Autodesk Fusion 360 part; units mm, degrees
(part 6 of 7)
sketch "Provisional CO PCB left-face seat sketch" plane through (0, 0, 24.5) normal (0, 0, 1) x (1, 0, 0) in component "Chamber / A3 top manifold with serial return"
  line L0 (4.9, 133) -> (8.95, 133)
  line L1 (8.95, 133) -> (8.95, 135)
  line L2 (8.95, 135) -> (4.9, 135)
  line L3 (4.9, 135) -> (4.9, 133)
  dimension "d2293" = 4.9
  dimension "d2294" = 133
  dimension "d2295" = 4.05
  dimension "d2296" = 2
  constraint horizontal L0
  constraint vertical L1
  constraint horizontal L2
  constraint vertical L3
  measures "d2293" horizontal distance of origin L0.start
  measures "d2294" vertical distance of origin L0.start
  measures "d2295" horizontal distance of L0.start L0.end
  measures "d2296" vertical distance of L0.end L1.end
extrude "Provisional CO PCB left-face seat" add sketch "Provisional CO PCB left-face seat sketch" along normal blind 2 bodies 74 in component "Chamber / A3 top manifold with serial return"
ref_plane "WorkPlane39" through (0, 0, 8) normal (0, 0, 1) x (1, 0, 0) in component "Chamber / A3 top manifold with serial return"
sketch "Provisional CO PCB left-face seat sketch (1)" plane through (0, 0, 8) normal (0, 0, 1) x (1, 0, 0) in component "Chamber / A3 top manifold with serial return"
  line L0 (4.9, 155) -> (8.95, 155)
  line L1 (8.95, 155) -> (8.95, 157)
  line L2 (8.95, 157) -> (4.9, 157)
  line L3 (4.9, 157) -> (4.9, 155)
  dimension "d2301" = 4.9
  dimension "d2302" = 155
  dimension "d2303" = 4.05
  dimension "d2304" = 2
  constraint horizontal L0
  constraint vertical L1
  constraint horizontal L2
  constraint vertical L3
  measures "d2301" horizontal distance of origin L0.start
  measures "d2302" vertical distance of origin L0.start
  measures "d2303" horizontal distance of L0.start L0.end
  measures "d2304" vertical distance of L0.end L1.end
extrude "Provisional CO PCB left-face seat (1)" add sketch "Provisional CO PCB left-face seat sketch (1)" along normal blind 2 bodies 74 in component "Chamber / A3 top manifold with serial return"
ref_plane "WorkPlane40" through (0, 0, 4.9) normal (0, 0, 1) x (1, 0, 0) in component "Chamber / A3 top manifold with serial return"
sketch "Provisional CO front-edge seat sketch" plane through (0, 0, 4.9) normal (0, 0, 1) x (1, 0, 0) in component "Chamber / A3 top manifold with serial return"
  line L0 (8.75, 133) -> (10.75, 133)
  line L1 (10.75, 133) -> (10.75, 135)
  line L2 (10.75, 135) -> (8.75, 135)
  line L3 (8.75, 135) -> (8.75, 133)
  dimension "d2309" = 8.75
  dimension "d2310" = 133
  dimension "d2311" = 2
  dimension "d2312" = 2
  constraint horizontal L0
  constraint vertical L1
  constraint horizontal L2
  constraint vertical L3
  measures "d2309" horizontal distance of origin L0.start
  measures "d2310" vertical distance of origin L0.start
  measures "d2311" horizontal distance of L0.start L0.end
  measures "d2312" vertical distance of L0.end L1.end
extrude "Provisional CO front-edge seat" add sketch "Provisional CO front-edge seat sketch" along normal blind 0.5 bodies 74 in component "Chamber / A3 top manifold with serial return"
ref_plane "WorkPlane41" through (0, 0, 6) normal (0, 0, 1) x (1, 0, 0) in component "Chamber / A3 top manifold with serial return"
sketch "Provisional CO upper corner keeper sketch" plane through (0, 0, 6) normal (0, 0, 1) x (1, 0, 0) in component "Chamber / A3 top manifold with serial return"
  line L0 (10.7, 155.5) -> (12.7, 155.5)
  line L1 (12.7, 155.5) -> (12.7, 159.5)
  line L2 (12.7, 159.5) -> (10.7, 159.5)
  line L3 (10.7, 159.5) -> (10.7, 155.5)
  dimension "d2317" = 10.7
  dimension "d2318" = 155.5
  dimension "d2319" = 2
  dimension "d2320" = 4
  constraint horizontal L0
  constraint vertical L1
  constraint horizontal L2
  constraint vertical L3
  measures "d2317" horizontal distance of origin L0.start
  measures "d2318" vertical distance of origin L0.start
  measures "d2319" horizontal distance of L0.start L0.end
  measures "d2320" vertical distance of L0.end L1.end
extrude "Provisional CO upper corner keeper" add sketch "Provisional CO upper corner keeper sketch" along normal blind 2 bodies 74 in component "Chamber / A3 top manifold with serial return"
ref_plane "WorkPlane42" through (0, 0, 25) normal (0, 0, 1) x (1, 0, 0) in component "Chamber / A3 top manifold with serial return"
sketch "Provisional CO lower corner keeper sketch" plane through (0, 0, 25) normal (0, 0, 1) x (1, 0, 0) in component "Chamber / A3 top manifold with serial return"
  line L0 (10.7, 131.5) -> (12.7, 131.5)
  line L1 (12.7, 131.5) -> (12.7, 134.3)
  line L2 (12.7, 134.3) -> (10.7, 134.3)
  line L3 (10.7, 134.3) -> (10.7, 131.5)
  dimension "d2325" = 10.7
  dimension "d2326" = 131.5
  dimension "d2327" = 2
  dimension "d2328" = 2.8
  constraint horizontal L0
  constraint vertical L1
  constraint horizontal L2
  constraint vertical L3
  measures "d2325" horizontal distance of origin L0.start
  measures "d2326" vertical distance of origin L0.start
  measures "d2327" horizontal distance of L0.start L0.end
  measures "d2328" vertical distance of L0.end L1.end
extrude "Provisional CO lower corner keeper" add sketch "Provisional CO lower corner keeper sketch" along normal blind 2 bodies 74 in component "Chamber / A3 top manifold with serial return"
ref_plane "WorkPlane43" through (0, 0, 4.9) normal (0, 0, 1) x (1, 0, 0) in component "Chamber / A3 top manifold with serial return"
sketch "Provisional MD62 front end-contact sketch" plane through (0, 0, 4.9) normal (0, 0, 1) x (1, 0, 0) in component "Chamber / A3 top manifold with serial return"
  line L0 (21.5, 164) -> (23.5, 164)
  line L1 (23.5, 164) -> (23.5, 166)
  line L2 (23.5, 166) -> (21.5, 166)
  line L3 (21.5, 166) -> (21.5, 164)
  dimension "d2333" = 21.5
  dimension "d2334" = 164
  dimension "d2335" = 2
  dimension "d2336" = 2
  constraint horizontal L0
  constraint vertical L1
  constraint horizontal L2
  constraint vertical L3
  measures "d2333" horizontal distance of origin L0.start
  measures "d2334" vertical distance of origin L0.start
  measures "d2335" horizontal distance of L0.start L0.end
  measures "d2336" vertical distance of L0.end L1.end
extrude "Provisional MD62 front end-contact" add sketch "Provisional MD62 front end-contact sketch" along normal blind 3.1 bodies 74 in component "Chamber / A3 top manifold with serial return"
ref_plane "WorkPlane7" through (0, 0, 27.3) normal (0, 0, 1) x (1, 0, 0) in component "Chamber / A3 four-screw service lid"
sketch "Sketch7" plane through (0, 0, 27.3) normal (0, 0, 1) x (1, 0, 0) in component "Chamber / A3 four-screw service lid"
  line L0 (21.5, 164) -> (23.5, 164)
  line L1 (23.5, 164) -> (23.5, 166)
  line L2 (23.5, 166) -> (21.5, 166)
  line L3 (21.5, 166) -> (21.5, 164)
  dimension "d2341" = 21.5
  dimension "d2342" = 164
  dimension "d2343" = 2
  dimension "d2344" = 2
  constraint horizontal L0
  constraint vertical L1
  constraint horizontal L2
  constraint vertical L3
  measures "d2341" horizontal distance of origin L0.start
  measures "d2342" vertical distance of origin L0.start
  measures "d2343" horizontal distance of L0.start L0.end
  measures "d2344" vertical distance of L0.end L1.end
extrude "Provisional MD62 rear end-stop — 0.3 mm gap" add sketch "Sketch7" along normal blind 8.8 bodies 75 in component "Chamber / A3 four-screw service lid"
ref_plane "WorkPlane44" through (0, 0, 4.9) normal (0, 0, 1) x (1, 0, 0) in component "Chamber / A3 top manifold with serial return"
sketch "Provisional MD62 front end-contact sketch (1)" plane through (0, 0, 4.9) normal (0, 0, 1) x (1, 0, 0) in component "Chamber / A3 top manifold with serial return"
  line L0 (21.5, 169.8) -> (23.5, 169.8)
  line L1 (23.5, 169.8) -> (23.5, 171.8)
  line L2 (23.5, 171.8) -> (21.5, 171.8)
  line L3 (21.5, 171.8) -> (21.5, 169.8)
  dimension "d2349" = 21.5
  dimension "d2350" = 169.8
  dimension "d2351" = 2
  dimension "d2352" = 2
  constraint horizontal L0
  constraint vertical L1
  constraint horizontal L2
  constraint vertical L3
  measures "d2349" horizontal distance of origin L0.start
  measures "d2350" vertical distance of origin L0.start
  measures "d2351" horizontal distance of L0.start L0.end
  measures "d2352" vertical distance of L0.end L1.end
extrude "Provisional MD62 front end-contact (1)" add sketch "Provisional MD62 front end-contact sketch (1)" along normal blind 3.1 bodies 74 in component "Chamber / A3 top manifold with serial return"
ref_plane "WorkPlane8" through (0, 0, 27.3) normal (0, 0, 1) x (1, 0, 0) in component "Chamber / A3 four-screw service lid"
sketch "Sketch8" plane through (0, 0, 27.3) normal (0, 0, 1) x (1, 0, 0) in component "Chamber / A3 four-screw service lid"
  line L0 (21.5, 169.8) -> (23.5, 169.8)
  line L1 (23.5, 169.8) -> (23.5, 171.8)
  line L2 (23.5, 171.8) -> (21.5, 171.8)
  line L3 (21.5, 171.8) -> (21.5, 169.8)
  dimension "d2357" = 21.5
  dimension "d2358" = 169.8
  dimension "d2359" = 2
  dimension "d2360" = 2
  constraint horizontal L0
  constraint vertical L1
  constraint horizontal L2
  constraint vertical L3
  measures "d2357" horizontal distance of origin L0.start
  measures "d2358" vertical distance of origin L0.start
  measures "d2359" horizontal distance of L0.start L0.end
  measures "d2360" vertical distance of L0.end L1.end
extrude "Provisional MD62 rear end-stop — 0.3 mm gap (1)" add sketch "Sketch8" along normal blind 8.8 bodies 75 in component "Chamber / A3 four-screw service lid"
ref_plane "WorkPlane45" through (0, 0, 4.9) normal (0, 0, 1) x (1, 0, 0) in component "Chamber / A3 top manifold with serial return"
sketch "Provisional MD62 lateral guide sketch" plane through (0, 0, 4.9) normal (0, 0, 1) x (1, 0, 0) in component "Chamber / A3 top manifold with serial return"
  line L0 (16.7, 163.5) -> (18.7, 163.5)
  line L1 (18.7, 163.5) -> (18.7, 171.5)
  line L2 (18.7, 171.5) -> (16.7, 171.5)
  line L3 (16.7, 171.5) -> (16.7, 163.5)
  dimension "d2365" = 16.7
  dimension "d2366" = 163.5
  dimension "d2367" = 2
  dimension "d2368" = 8
  constraint horizontal L0
  constraint vertical L1
  constraint horizontal L2
  constraint vertical L3
  measures "d2365" horizontal distance of origin L0.start
  measures "d2366" vertical distance of origin L0.start
  measures "d2367" horizontal distance of L0.start L0.end
  measures "d2368" vertical distance of L0.end L1.end
extrude "Provisional MD62 lateral guide" add sketch "Provisional MD62 lateral guide sketch" along normal blind 5.1 bodies 74 in component "Chamber / A3 top manifold with serial return"
ref_plane "WorkPlane46" through (0, 0, 4.9) normal (0, 0, 1) x (1, 0, 0) in component "Chamber / A3 top manifold with serial return"
sketch "Provisional MD62 lateral guide sketch (1)" plane through (0, 0, 4.9) normal (0, 0, 1) x (1, 0, 0) in component "Chamber / A3 top manifold with serial return"
  line L0 (33.3, 163.5) -> (35.3, 163.5)
  line L1 (35.3, 163.5) -> (35.3, 171.5)
  line L2 (35.3, 171.5) -> (33.3, 171.5)
  line L3 (33.3, 171.5) -> (33.3, 163.5)
  dimension "d2373" = 33.3
  dimension "d2374" = 163.5
  dimension "d2375" = 2
  dimension "d2376" = 8
  constraint horizontal L0
  constraint vertical L1
  constraint horizontal L2
  constraint vertical L3
  measures "d2373" horizontal distance of origin L0.start
  measures "d2374" vertical distance of origin L0.start
  measures "d2375" horizontal distance of L0.start L0.end
  measures "d2376" vertical distance of L0.end L1.end
extrude "Provisional MD62 lateral guide (1)" add sketch "Provisional MD62 lateral guide sketch (1)" along normal blind 5.1 bodies 74 in component "Chamber / A3 top manifold with serial return"
ref_plane "WorkPlane47" through (0, 0, 4.9) normal (0, 0, 1) x (1, 0, 0) in component "Chamber / A3 top manifold with serial return"
sketch "Provisional humidity PCB foot sketch" plane through (0, 0, 4.9) normal (0, 0, 1) x (1, 0, 0) in component "Chamber / A3 top manifold with serial return"
  line L0 (54, 164) -> (56, 164)
  line L1 (56, 164) -> (56, 166)
  line L2 (56, 166) -> (54, 166)
  line L3 (54, 166) -> (54, 164)
  dimension "d2381" = 54
  dimension "d2382" = 164
  dimension "d2383" = 2
  dimension "d2384" = 2
  constraint horizontal L0
  constraint vertical L1
  constraint horizontal L2
  constraint vertical L3
  measures "d2381" horizontal distance of origin L0.start
  measures "d2382" vertical distance of origin L0.start
  measures "d2383" horizontal distance of L0.start L0.end
  measures "d2384" vertical distance of L0.end L1.end
extrude "Provisional humidity PCB foot" add sketch "Provisional humidity PCB foot sketch" along normal blind 1.1 bodies 74 in component "Chamber / A3 top manifold with serial return"
ref_plane "WorkPlane48" through (0, 0, 4.9) normal (0, 0, 1) x (1, 0, 0) in component "Chamber / A3 top manifold with serial return"
sketch "Provisional humidity PCB foot sketch (1)" plane through (0, 0, 4.9) normal (0, 0, 1) x (1, 0, 0) in component "Chamber / A3 top manifold with serial return"
  line L0 (67, 172) -> (69, 172)
  line L1 (69, 172) -> (69, 174)
  line L2 (69, 174) -> (67, 174)
  line L3 (67, 174) -> (67, 172)
  dimension "d2389" = 67
  dimension "d2390" = 172
  dimension "d2391" = 2
  dimension "d2392" = 2
  constraint horizontal L0
  constraint vertical L1
  constraint horizontal L2
  constraint vertical L3
  measures "d2389" horizontal distance of origin L0.start
  measures "d2390" vertical distance of origin L0.start
  measures "d2391" horizontal distance of L0.start L0.end
  measures "d2392" vertical distance of L0.end L1.end
extrude "Provisional humidity PCB foot (1)" add sketch "Provisional humidity PCB foot sketch (1)" along normal blind 1.1 bodies 74 in component "Chamber / A3 top manifold with serial return"
ref_plane "WorkPlane49" through (0, 0, 7.9) normal (0, 0, 1) x (1, 0, 0) in component "Chamber / A3 top manifold with serial return"
sketch "Provisional humidity corner keeper sketch" plane through (0, 0, 7.9) normal (0, 0, 1) x (1, 0, 0) in component "Chamber / A3 top manifold with serial return"
  line L0 (68, 164) -> (70.6, 164)
  line L1 (70.6, 164) -> (70.6, 166)
  line L2 (70.6, 166) -> (68, 166)
  line L3 (68, 166) -> (68, 164)
  dimension "d2397" = 68
  dimension "d2398" = 164
  dimension "d2399" = 2.6
  dimension "d2400" = 2
  constraint horizontal L0
  constraint vertical L1
  constraint horizontal L2
  constraint vertical L3
  measures "d2397" horizontal distance of origin L0.start
  measures "d2398" vertical distance of origin L0.start
  measures "d2399" horizontal distance of L0.start L0.end
  measures "d2400" vertical distance of L0.end L1.end
extrude "Provisional humidity corner keeper" add sketch "Provisional humidity corner keeper sketch" along normal blind 2 bodies 74 in component "Chamber / A3 top manifold with serial return"
component "01 Shape A housing" placed x (1, 0, 0) y (0, 1, 0) z (0, 0, 1) at (0, 0, 0)
component "02 Single rear cover" placed x (1, 0, 0) y (0, 1, 0) z (0, 0, 1) at (0, 0, 0)
component "03 Guition factory casing — measured envelope" placed x (1, 0, 0) y (0, 1, 0) z (0, 0, 1) at (0, 0, 0)
component "04 Guition front glass — drawing reference" placed x (1, 0, 0) y (0, 1, 0) z (0, 0, 1) at (0, 0, 0)
component "05 Active 4.3 inch screen" placed x (1, 0, 0) y (0, 1, 0) z (0, 0, 1) at (0, 0, 0)
component "06 Guition PCB and connectors — illustrative detail" placed x (1, 0, 0) y (0, 1, 0) z (0, 0, 1) at (0, 0, 0)
component "M3 x 8 button screw — GEN-M3-BHCS-L8-AF2" placed x (1, 0, 0) y (0, 1, 0) z (0, 0, 1) at (8, 8, 41.35)
component "M3 insert OD4.2 x5 — GEN-M3-HEATSET-OD4.2-L5" placed x (1, 0, 0) y (0, 1, 0) z (0, 0, 1) at (8, 8, 39)
component "Carrier / removable electronics tray" placed x (1, 0, 0) y (0, 1, 0) z (0, 0, 1) at (0, 0, 0)
component "Carrier / future PCB allocation — layout pending" placed x (1, 0, 0) y (0, 1, 0) z (0, 0, 1) at (0, 0, 0)
component "M2 x 7 socket_cap screw — GEN-M2-SHCS-L7-AF1.5" placed x (1, 0, 0) y (0, 1, 0) z (0, 0, 1) at (76, 28, 22.1)
component "M2 insert OD3.2 x4 — GEN-M2-HEATSET-OD3.2-L4" placed x (1, 0, 0) y (0, 1, 0) z (0, 0, 1) at (76, 28, 18.5)
component "Display / lower rear-release retainer" placed x (1, 0, 0) y (0, 1, 0) z (0, 0, 1) at (0, 0, 0)
component "Display / upper rear-release retainer" placed x (1, 0, 0) y (0, 1, 0) z (0, 0, 1) at (0, 0, 0)
component "M2 x 5 socket_cap screw — GEN-M2-SHCS-L5-AF1.5" placed x (1, 0, 0) y (0, 1, 0) z (0, 0, 1) at (69, 12.3, 20.5)
component "Battery / FMA protected holder - owner-measured envelope" placed x (1, 0, 0) y (0, 1, 0) z (0, 0, 1) at (0, 0, 0)
component "Battery / 18650 cell A - owner-rated 3400 mAh" placed x (1, 0, 0) y (0, 1, 0) z (0, 0, 1) at (0, 0, 0)
component "Battery / 18650 cell B - owner-rated 3400 mAh" placed x (1, 0, 0) y (0, 1, 0) z (0, 0, 1) at (0, 0, 0)
component "Battery / red RCY disconnect body - provisional reference" placed x (1, 0, 0) y (0, 1, 0) z (0, 0, 1) at (0, 0, 0)
component "Battery / red RCY disconnect mate - provisional reference" placed x (1, 0, 0) y (0, 1, 0) z (0, 0, 1) at (0, 0, 0)
component "Controls / left 1NO button body" placed x (1, 0, 0) y (0, 1, 0) z (0, 0, 1) at (0, 0, 0)
component "Controls / left momentary power cap" placed x (1, 0, 0) y (0, 1, 0) z (0, 0, 1) at (0, 0, 0)
component "Controls / button retaining nut reference" placed x (1, 0, 0) y (0, 1, 0) z (0, 0, 1) at (0, 0, 0)
component "USB A3 — tiny flush metal bezel and hidden flange" placed x (1, 0, 0) y (0, 1, 0) z (0, 0, 1) at (0, 0, 0)
component "USB A3 — removable printed support frame" placed x (1, 0, 0) y (0, 1, 0) z (0, 0, 1) at (0, 0, 0)
component "USB A3 — hidden metal retaining bridge" placed x (1, 0, 0) y (0, 1, 0) z (0, 0, 1) at (0, 0, 0)
component "USB A3 — supported 0.60 mm daughterboard provisional" placed x (1, 0, 0) y (0, 1, 0) z (0, 0, 1) at (0, 0, 0)
component "USB A3 — GCT USB4720 shell drawing reconstruction" placed x (1, 0, 0) y (0, 1, 0) z (0, 0, 1) at (0, 0, 0)
component "USB A3 — tongue and rear insulator reference" placed x (1, 0, 0) y (0, 1, 0) z (0, 0, 1) at (0, 0, 0)
component "USB A3 — GCT LIM gasket nominal reference" placed x (1, 0, 0) y (0, 1, 0) z (0, 0, 1) at (0, 0, 0)
component "USB A3 — illustrative contact stripes" placed x (1, 0, 0) y (0, 1, 0) z (0, 0, 1) at (0, 0, 0)
component "Chamber / A3 top manifold with serial return" placed x (1, 0, 0) y (0, 1, 0) z (0, 0, 1) at (0, 0, 0)
component "Chamber / A3 four-screw service lid" placed x (1, 0, 0) y (0, 1, 0) z (0, 0, 1) at (0, 0, 0)
component "Chamber / AO2 hand-tight adapter reference" placed x (1, 0, 0) y (0, 1, 0) z (0, 0, 1) at (0, 0, 0)
component "Sensor / AO2 dry body with wetted threaded nose" placed x (1, 0, 0) y (0, 1, 0) z (0, 0, 1) at (0, 0, 0)
component "Sensor / AO2 cable connector allowance" placed x (1, 0, 0) y (0, 1, 0) z (0, 0, 1) at (0, 0, 0)
component "Sensor / ZE07-CO drawing-derived assembly" placed x (1, 0, 0) y (0, 1, 0) z (0, 0, 1) at (0, 0, 0)
component "Sensor / MD62 body and full-length lead references" placed x (1, 0, 0) y (0, 1, 0) z (0, 0, 1) at (0, 0, 0)
component "Sensor / GYBMEP humidity breakout reference" placed x (1, 0, 0) y (0, 1, 0) z (0, 0, 1) at (0, 0, 0)
component "Gas / Viewer-left inlet fitting reference" placed x (1, 0, 0) y (0, 1, 0) z (0, 0, 1) at (0, 0, 0)
component "Gas / Viewer-right exhaust fitting reference" placed x (1, 0, 0) y (0, 1, 0) z (0, 0, 1) at (0, 0, 0)
component "Chamber / AO2 face-seal allowance" placed x (1, 0, 0) y (0, 1, 0) z (0, 0, 1) at (0, 0, 0)
component "Chamber / sealed harness feedthrough allowance" placed x (1, 0, 0) y (0, 1, 0) z (0, 0, 1) at (0, 0, 0)
component "M3 x 8 button screw — GEN-M3-BHCS-L8-AF2" placed x (1, 0, 0) y (0, 1, 0) z (0, 0, 1) at (77, 8, 41.35)
component "M3 x 8 button screw — GEN-M3-BHCS-L8-AF2" placed x (1, 0, 0) y (0, 1, 0) z (0, 0, 1) at (8, 172, 41.35)
component "M3 x 8 button screw — GEN-M3-BHCS-L8-AF2" placed x (1, 0, 0) y (0, 1, 0) z (0, 0, 1) at (77, 172, 41.35)
component "M3 insert OD4.2 x5 — GEN-M3-HEATSET-OD4.2-L5" placed x (1, 0, 0) y (0, 1, 0) z (0, 0, 1) at (77, 8, 39)
component "M3 insert OD4.2 x5 — GEN-M3-HEATSET-OD4.2-L5" placed x (1, 0, 0) y (0, 1, 0) z (0, 0, 1) at (8, 172, 39)
component "M3 insert OD4.2 x5 — GEN-M3-HEATSET-OD4.2-L5" placed x (1, 0, 0) y (0, 1, 0) z (0, 0, 1) at (77, 172, 39)
component "M2 x 7 socket_cap screw — GEN-M2-SHCS-L7-AF1.5" placed x (1, 0, 0) y (0, 1, 0) z (0, 0, 1) at (54.8, 114, 22.1)
component "M2 insert OD3.2 x4 — GEN-M2-HEATSET-OD3.2-L4" placed x (1, 0, 0) y (0, 1, 0) z (0, 0, 1) at (54.8, 114, 18.5)
component "M2 x 5 socket_cap screw — GEN-M2-SHCS-L5-AF1.5" placed x (1, 0, 0) y (0, 1, 0) z (0, 0, 1) at (10.5, 126, 20.5)
component "M2 insert OD3.2 x4 — GEN-M2-HEATSET-OD3.2-L4" placed x (1, 0, 0) y (0, 1, 0) z (0, 0, 1) at (69, 12.3, 18.5)
component "M2 insert OD3.2 x4 — GEN-M2-HEATSET-OD3.2-L4" placed x (1, 0, 0) y (0, 1, 0) z (0, 0, 1) at (10.5, 126, 18.5)
component "M2 x 5 socket_cap screw — GEN-M2-SHCS-L5-AF1.5" placed x (1, 0, 0) y (0, 1, 0) z (0, 0, 1) at (33.25, 18.25, 33.2)
component "M2 x 5 socket_cap screw — GEN-M2-SHCS-L5-AF1.5" placed x (1, 0, 0) y (0, 1, 0) z (0, 0, 1) at (51.75, 18.25, 33.2)
component "M2 insert OD3.2 x4 — GEN-M2-HEATSET-OD3.2-L4" placed x (1, 0, 0) y (0, 1, 0) z (0, 0, 1) at (33.25, 18.25, 31.2)
component "M2 insert OD3.2 x4 — GEN-M2-HEATSET-OD3.2-L4" placed x (1, 0, 0) y (0, 1, 0) z (0, 0, 1) at (51.75, 18.25, 31.2)
component "M2 x 5 socket_cap screw — GEN-M2-SHCS-L5-AF1.5" placed x (1, 0, 0) y (0, 1, 0) z (0, 0, 1) at (18, 159, 38)
component "M2 x 5 socket_cap screw — GEN-M2-SHCS-L5-AF1.5" placed x (1, 0, 0) y (0, 1, 0) z (0, 0, 1) at (30.5, 135, 38)
component "M2 x 5 socket_cap screw — GEN-M2-SHCS-L5-AF1.5" placed x (1, 0, 0) y (0, 1, 0) z (0, 0, 1) at (17, 172.2, 38)
component "M2 x 5 socket_cap screw — GEN-M2-SHCS-L5-AF1.5" placed x (1, 0, 0) y (0, 1, 0) z (0, 0, 1) at (68, 172.2, 38)
component "M2 insert OD3.2 x4 — GEN-M2-HEATSET-OD3.2-L4" placed x (1, 0, 0) y (0, 1, 0) z (0, 0, 1) at (18, 159, 36)
component "M2 insert OD3.2 x4 — GEN-M2-HEATSET-OD3.2-L4" placed x (1, 0, 0) y (0, 1, 0) z (0, 0, 1) at (30.5, 135, 36)
component "M2 insert OD3.2 x4 — GEN-M2-HEATSET-OD3.2-L4" placed x (1, 0, 0) y (0, 1, 0) z (0, 0, 1) at (17, 172.2, 36)
component "M2 insert OD3.2 x4 — GEN-M2-HEATSET-OD3.2-L4" placed x (1, 0, 0) y (0, 1, 0) z (0, 0, 1) at (68, 172.2, 36)
component "Trimix_Enclosure_A3 v2" placed x (1, 0, 0) y (0, 1, 0) z (0, 0, 1) at (0, 0, 0) in component "03 Guition factory casing — measured envelope"
component "01 Shape A housing" placed x (1, 0, 0) y (0, 1, 0) z (0, 0, 1) at (0, 0, 0) in component "Chamber / A3 four-screw service lid"
equation "CaseWidth = 85 mm" comment "Accepted maximum starting width; test narrower packaging"
equation "CaseHeight = 180 mm" comment "Taller top sampling pod accepted for a slimmer grip"
equation "CaseDepth = 43 mm" comment "Body including flush rear screw heads"
equation "Wall = 2.4 mm" comment "Nominal printed structural wall, selected sections minimum2mm"
equation "RearInset = 0.25 mm" comment "Small rearward taper per side; Shape A straight-sided intent"
equation "CornerRadius = 8 mm" comment "Restrained Shape A outline rounds"
equation "Cover = 2.4 mm" comment "Single rear cover nominal thickness"
equation "CoverGap = 0.2 mm" comment "Assembly gap, not a qualified weather seal"
equation "DisplayWidth = 69.3 mm" comment "Owner measured retained factory casing"
equation "DisplayHeight = 116.8 mm" comment "Owner measured retained factory casing"
equation "DisplayDepth = 13.7 mm" comment "Owner measured with factory back removed"
equation "DisplayX = ( CaseWidth - DisplayWidth ) / 2" comment "Purchased assembly remains centred"
equation "DisplayY = 5.2 mm" comment "Fixed lower front border"
equation "DisplayFront = 0.4 mm" comment "Front recess"
equation "DisplayFit = 0.4 mm" comment "Provisional fit clearance per side"
equation "GlassWidth = 66.8 mm" comment "Manufacturer drawing reference"
equation "GlassHeight = 114.4 mm" comment "Manufacturer drawing reference"
equation "ActiveWidth = 56.16 mm" comment "Manufacturer active-area reference"
equation "ActiveHeight = 93.60 mm" comment "Manufacturer active-area reference"
equation "HolderWidth = 42 mm" comment "Owner measured occupied protected FMA holder"
equation "HolderHeight = 80.4 mm" comment "Owner measured occupied protected FMA holder"
equation "HolderDepth = 20.35 mm" comment "Owner measured occupied protected FMA holder"
equation "HolderX = 5.4 mm" comment "Right-hand rear battery bay"
equation "HolderY = 27 mm" comment "Clear bottom USB cartridge and cable region"
equation "HolderZ = 16.5 mm" comment "2.4mm beyond maximum purchased display depth"
equation "PcbX = 50.4 mm" comment "PCB strip beside holder; no stack behind battery"
equation "PcbY = 21 mm" comment "Low end of PCB strip"
equation "PcbWidth = CaseWidth - PcbX - 4.6 mm" comment "Future PCB allocation; routed fit pending"
equation "PcbHeight = 99 mm" comment "Future PCB strip height before button notch"
equation "PcbZ = 20.5 mm" comment "PCB front plane; carrier and support below"
equation "ButtonY = 113 mm" comment "Viewer-left button above pack; PCB notch"
equation "ButtonZ = 31 mm" comment "Unmeasured button assembly depth centre"
equation "UsbX = CaseWidth / 2" comment "Centred bottom USB socket"
equation "UsbZ = 26 mm" comment "Bottom USB socket depth centre"
equation "GasY = CaseHeight - 17.5 mm" comment "Upper opposed sample ports"
equation "GasZ = 22 mm" comment "Sample port depth centre"
equation "d39 = CaseWidth"
equation "d40 = CaseHeight"
equation "d41 = CaseDepth - Cover"
equation "d43 = RearInset"
equation "d44 = RearInset"
equation "d45 = CaseWidth - 2 * RearInset"
equation "d46 = CaseHeight - 2 * RearInset"
equation "d48 = CornerRadius"
equation "d51 = Wall"
equation "d52 = Wall"
equation "d53 = CaseWidth - 2 * Wall"
equation "d54 = CaseHeight - 2 * Wall"
equation "d55 = CaseDepth"
equation "d58 = CornerRadius - Wall"
equation "d59 = Wall"
equation "d61 = Wall"
equation "d63 = CaseWidth - 2 * Wall"
equation "d64 = CaseHeight - Wall - 128 mm"
equation "d65 = CaseDepth"
equation "d68 = CornerRadius - Wall"
equation "d71 = DisplayX - DisplayFit"
equation "d72 = DisplayY - DisplayFit"
equation "d73 = DisplayWidth + 2 * DisplayFit"
equation "d74 = DisplayHeight + 2 * DisplayFit"
equation "d81 = -( -( GasZ ) )"
equation "d82 = GasY"
equation "d84 = CaseWidth + 2 mm"
equation "d86 = CaseWidth - Wall - 1 mm"
equation "d88 = -( -( ButtonZ ) )"
equation "d89 = ButtonY"
equation "d91 = Wall + 2 mm"
equation "d93 = CaseDepth - Cover + CoverGap"
equation "d95 = RearInset"
equation "d96 = RearInset"
equation "d97 = CaseWidth - 2 * RearInset"
equation "d98 = CaseHeight - 2 * RearInset"
equation "d99 = Cover - CoverGap"
equation "d102 = CornerRadius"
equation "d105 = DisplayFront"
equation "d107 = DisplayX"
equation "d108 = DisplayY"
equation "d109 = DisplayWidth"
equation "d110 = DisplayHeight"
equation "d111 = DisplayDepth"
equation "d115 = DisplayFront + 3 mm"
equation "d117 = DisplayX + ( DisplayWidth - 65.4 mm ) / 2"
equation "d118 = DisplayY + ( DisplayHeight - 108 mm ) / 2"
equation "d123 = DisplayFront - 0.1 mm"
equation "d125 = DisplayX + ( DisplayWidth - GlassWidth ) / 2"
equation "d126 = DisplayY + ( DisplayHeight - GlassHeight ) / 2"
equation "d127 = GlassWidth"
equation "d128 = GlassHeight"
equation "d131 = DisplayFront"
equation "d133 = DisplayX + ( DisplayWidth - GlassWidth ) / 2"
equation "d134 = DisplayY + ( DisplayHeight - GlassHeight ) / 2"
equation "d135 = GlassWidth"
equation "d136 = GlassHeight"
equation "d139 = DisplayFront - 0.1 mm"
equation "d141 = DisplayX + ( DisplayWidth - ActiveWidth ) / 2"
equation "d142 = DisplayY + ( DisplayHeight - ActiveHeight ) / 2"
equation "d143 = ActiveWidth"
equation "d144 = ActiveHeight"
equation "d147 = DisplayFront"
equation "d149 = DisplayX + ( DisplayWidth - ActiveWidth ) / 2"
equation "d150 = DisplayY + ( DisplayHeight - ActiveHeight ) / 2"
equation "d151 = ActiveWidth"
equation "d152 = ActiveHeight"
equation "d157 = DisplayX + ( DisplayWidth - 65.06 mm ) / 2"
equation "d158 = DisplayY + ( DisplayHeight - 108 mm ) / 2"
equation "d165 = DisplayX + 4.65 mm"
equation "d166 = DisplayY + 7.1 mm"
equation "d172 = DisplayX + 4.65 mm"
equation "d173 = DisplayY + 109.7 mm"
equation "d179 = DisplayX + 64.65 mm"
equation "d180 = DisplayY + 7.1 mm"
equation "d186 = DisplayX + 64.65 mm"
equation "d187 = DisplayY + 109.7 mm"
equation "d193 = DisplayX + 12.15 mm"
equation "d194 = DisplayY + 70.9 mm"
equation "d201 = DisplayX + 44.15 mm"
equation "d202 = DisplayY + 85.9 mm"
equation "d209 = DisplayX + 31.15 mm"
equation "d210 = DisplayY + 74.9 mm"
equation "d217 = DisplayX + 11.15 mm"
equation "d218 = DisplayY + 13.9 mm"
equation "d225 = DisplayX + 21.15 mm"
equation "d226 = DisplayY + 18.9 mm"
equation "d233 = DisplayX + 27.15 mm"
equation "d234 = DisplayY + 4.9 mm"
equation "d241 = DisplayX + 20.15 mm"
equation "d242 = DisplayY + 57.9 mm"
equation "d249 = DisplayX + 49.15 mm"
equation "d250 = DisplayY + 29.9 mm"
equation "d255 = CaseDepth - 13 mm"
equation "d257 = ( 8 mm ) - 3.7 mm"
equation "d258 = Wall - 0.1 mm"
equation "d263 = CaseDepth - 13 mm"
equation "d270 = CaseDepth - 9 mm"
equation "d277 = CaseDepth - 3.8 mm"
equation "d284 = CaseDepth - 3.9 mm"
equation "d291 = CaseDepth - 1.65 mm"
equation "d298 = CaseDepth - 3.9 mm"
equation "d305 = CaseDepth - 13 mm"
equation "d307 = ( CaseWidth - 8 mm ) - 3.7 mm"
equation "d308 = Wall - 0.1 mm"
equation "d313 = CaseDepth - 13 mm"
equation "d315 = CaseWidth - 8 mm"
equation "d320 = CaseDepth - 9 mm"
equation "d322 = CaseWidth - 8 mm"
equation "d327 = CaseDepth - 3.8 mm"
equation "d329 = CaseWidth - 8 mm"
equation "d334 = CaseDepth - 3.9 mm"
equation "d336 = CaseWidth - 8 mm"
equation "d341 = CaseDepth - 1.65 mm"
equation "d343 = CaseWidth - 8 mm"
equation "d348 = CaseDepth - 3.9 mm"
equation "d350 = CaseWidth - 8 mm"
equation "d355 = CaseDepth - 13 mm"
equation "d357 = ( 8 mm ) - 3.7 mm"
equation "d358 = CaseHeight - 11.5 mm"
equation "d363 = CaseDepth - 13 mm"
equation "d366 = CaseHeight - 8 mm"
equation "d370 = CaseDepth - 9 mm"
equation "d373 = CaseHeight - 8 mm"
equation "d377 = CaseDepth - 3.8 mm"
equation "d380 = CaseHeight - 8 mm"
equation "d384 = CaseDepth - 3.9 mm"
equation "d387 = CaseHeight - 8 mm"
equation "d391 = CaseDepth - 1.65 mm"
equation "d394 = CaseHeight - 8 mm"
equation "d398 = CaseDepth - 3.9 mm"
equation "d401 = CaseHeight - 8 mm"
equation "d405 = CaseDepth - 13 mm"
equation "d407 = ( CaseWidth - 8 mm ) - 3.7 mm"
equation "d408 = CaseHeight - 10.5 mm"
equation "d413 = CaseDepth - 13 mm"
equation "d415 = CaseWidth - 8 mm"
equation "d416 = CaseHeight - 8 mm"
equation "d420 = CaseDepth - 9 mm"
equation "d422 = CaseWidth - 8 mm"
equation "d423 = CaseHeight - 8 mm"
equation "d427 = CaseDepth - 3.8 mm"
equation "d429 = CaseWidth - 8 mm"
equation "d430 = CaseHeight - 8 mm"
equation "d434 = CaseDepth - 3.9 mm"
equation "d436 = CaseWidth - 8 mm"
equation "d437 = CaseHeight - 8 mm"
equation "d441 = CaseDepth - 1.65 mm"
equation "d443 = CaseWidth - 8 mm"
equation "d444 = CaseHeight - 8 mm"
equation "d448 = CaseDepth - 3.9 mm"
equation "d450 = CaseWidth - 8 mm"
equation "d451 = CaseHeight - 8 mm"
equation "d493 = CaseDepth - Cover - 2 mm"
equation "d495 = Wall + 0.25 mm"
equation "d501 = CaseDepth - Cover - 2 mm"
equation "d503 = Wall + 0.25 mm"
equation "d509 = CaseDepth - Cover - 2 mm"
equation "d511 = CaseWidth - Wall - 2.25 mm"
equation "d517 = CaseDepth - Cover - 2 mm"
equation "d519 = CaseWidth - Wall - 2.25 mm"
equation "d527 = Wall - 0.1 mm"
equation "d529 = 50.2 mm - Wall + 0.1 mm"
equation "d543 = ( CaseWidth - 9 mm ) - 3.6 mm"
equation "d544 = ( 28 mm ) - 3.6 mm"
equation "d545 = CaseWidth - Wall + 0.1 mm - ( ( CaseWidth - 9 mm ) - 3.6 mm )"
equation "d551 = CaseWidth - 9 mm"
equation "d559 = ( 114 mm ) - 3.6 mm"
equation "d573 = PcbX - 0.2 mm"
equation "d574 = PcbY - 0.5 mm"
equation "d575 = PcbWidth + 0.4 mm"
equation "d576 = PcbHeight + 1 mm"
equation "d579 = PcbZ"
equation "d581 = PcbX"
equation "d582 = PcbY"
equation "d583 = PcbWidth"
equation "d584 = PcbHeight"
equation "d589 = CaseWidth - 26 mm"
equation "d597 = CaseWidth - 9 mm"
equation "d611 = CaseWidth - 26 mm"
equation "d619 = CaseWidth - 9 mm"
equation "d631 = PcbZ + 1.6 mm"
equation "d639 = PcbZ + 1.6 mm"
equation "d647 = PcbZ + 1.6 mm"
equation "d695 = CaseWidth - 17.7 mm"
equation "d703 = CaseWidth - 16 mm"
equation "d710 = CaseWidth - 16 mm"
equation "d717 = DisplayX + 2.65 mm"
equation "d724 = DisplayX + 2.65 mm"
equation "d731 = ( CaseWidth - 16 mm ) - 3.5 mm"
equation "d739 = ( CaseWidth - 16 mm ) - 3 mm"
equation "d740 = DisplayY + 0.5 mm"
equation "d747 = CaseWidth - 16 mm"
equation "d754 = DisplayX - 0.85 mm"
equation "d762 = DisplayX + 0.65 mm"
equation "d763 = DisplayY + DisplayHeight - 2.2 mm"
equation "d770 = DisplayX + 2.65 mm"
equation "d791 = HolderZ"
equation "d793 = HolderX"
equation "d794 = HolderY"
equation "d795 = HolderWidth"
equation "d796 = HolderHeight"
equation "d797 = HolderDepth"
equation "d801 = HolderZ + 1.1 mm"
equation "d803 = HolderX + 1 mm"
equation "d804 = HolderY + 2 mm"
equation "d805 = HolderWidth - 2 mm"
equation "d806 = HolderHeight - 4 mm"
equation "d807 = HolderDepth"
equation "d809 = HolderY + 5 mm"
equation "d811 = HolderX + 10.8 mm"
equation "d812 = -( -( HolderZ + 10.25 mm ) )"
equation "d816 = HolderY + 5 mm"
equation "d818 = HolderX + 31.2 mm"
equation "d819 = -( -( HolderZ + 10.25 mm ) )"
equation "d849 = Wall - 0.1 mm"
equation "d850 = HolderY"
equation "d851 = HolderX - Wall - 0.4 mm"
equation "d852 = HolderHeight"
equation "d857 = Wall - 0.1 mm"
equation "d858 = HolderY - 2.5 mm"
equation "d859 = 50.2 mm - Wall + 0.1 mm"
equation "d865 = Wall - 0.1 mm"
equation "d866 = HolderY + HolderHeight + 0.5 mm"
equation "d867 = 50.2 mm - Wall + 0.1 mm"
equation "d873 = HolderX"
equation "d874 = HolderY"
equation "d876 = HolderHeight"
equation "d879 = HolderZ + HolderDepth + 0.5 mm"
equation "d881 = HolderX"
equation "d882 = HolderY + 12 mm"
equation "d885 = CaseDepth - Cover + CoverGap - HolderZ - HolderDepth - 0.5 mm + 0.2 mm"
equation "d889 = HolderX + HolderWidth - 2 mm"
equation "d890 = HolderY"
equation "d892 = HolderHeight"
equation "d895 = HolderZ + HolderDepth + 0.5 mm"
equation "d897 = HolderX + HolderWidth - 2 mm"
equation "d898 = HolderY + 12 mm"
equation "d901 = CaseDepth - Cover + CoverGap - HolderZ - HolderDepth - 0.5 mm + 0.2 mm"
equation "d903 = CaseWidth - 18 mm"
equation "d905 = -( -( ButtonZ ) )"
equation "d906 = ButtonY"
equation "d910 = CaseWidth"
equation "d912 = -( -( ButtonZ ) )"
equation "d913 = ButtonY"
equation "d917 = CaseWidth - 25 mm"
equation "d919 = -( -( ( ButtonZ - 4 mm ) + ( 8 mm ) ) )"
equation "d920 = ButtonY - 4 mm"
equation "d925 = CaseWidth + 1.3 mm"
equation "d927 = -( -( ButtonZ ) )"
equation "d928 = ButtonY"
equation "d932 = CaseWidth - 4.5 mm"
equation "d934 = -( -( ButtonZ ) )"
equation "d935 = ButtonY"
equation "d939 = CaseWidth - 4.6 mm"
equation "d941 = -( -( ButtonZ ) )"
equation "d942 = ButtonY"
equation "d948 = PcbX - 0.2 mm"
equation "d950 = UsbX + 13.9 mm - PcbX"
equation "d956 = PcbX - 0.2 mm"
equation "d958 = UsbX + 13.9 mm - PcbX"
equation "d962 = CaseDepth - 10 mm"
equation "d969 = CaseDepth - 10 mm"
equation "d972 = CaseHeight - 8 mm"
equation "d976 = CaseDepth - 10 mm"
equation "d978 = CaseWidth - 8 mm"
equation "d983 = CaseDepth - 10 mm"
equation "d985 = CaseWidth - 8 mm"
equation "d986 = CaseHeight - 8 mm"
equation "d992 = UsbX - ( 7 mm )"
equation "d993 = -( -( ( UsbZ - ( 4 mm ) ) + ( 8 mm ) ) )"
equation "d1002 = UsbX - 10 mm"
equation "d1003 = -( -( ( UsbZ - 5 mm ) + ( 11 mm ) ) )"
equation "d1010 = UsbX - 6.5 mm"
equation "d1011 = -( -( ( UsbZ - 3.5 mm ) + ( 7 mm ) ) )"
equation "d1018 = UsbX - ( 4.22 mm )"
equation "d1019 = -( -( ( UsbZ - ( 1.33 mm ) ) + ( 2.66 mm ) ) )"
equation "d1028 = UsbX - ( 4.57 mm )"
equation "d1029 = -( -( ( UsbZ - ( 1.675 mm ) ) + ( 3.35 mm ) ) )"
equation "d1038 = UsbX - ( 4.82 mm )"
equation "d1039 = -( -( ( UsbZ - ( 1.93 mm ) ) + ( 3.86 mm ) ) )"
equation "d1048 = UsbX - ( 4.419249488 mm )"
equation "d1049 = -( -( ( UsbZ - ( 1.529249488 mm ) ) + ( 3.058498976 mm ) ) )"
equation "d1058 = UsbX - ( 4.22 mm )"
equation "d1059 = -( -( ( UsbZ - ( 1.33 mm ) ) + ( 2.66 mm ) ) )"
equation "d1066 = UsbZ - 7 mm"
equation "d1068 = UsbX - 12.9 mm"
equation "d1074 = UsbZ - 5 mm"
equation "d1076 = UsbX - 12.9 mm"
equation "d1082 = UsbZ - 3.2 mm"
equation "d1084 = UsbX - 6.5 mm"
equation "d1090 = UsbZ - 7 mm"
equation "d1092 = UsbX - 9.25 mm"
equation "d1097 = UsbZ + 0.95 mm"
equation "d1099 = UsbX - 9.25 mm"
equation "d1104 = UsbZ - 7 mm"
equation "d1106 = UsbX + 9.25 mm"
equation "d1111 = UsbZ + 0.95 mm"
equation "d1113 = UsbX + 9.25 mm"
equation "d1118 = UsbZ - 5 mm"
equation "d1120 = UsbX - 5.1 mm"
equation "d1126 = UsbZ - 5 mm"
equation "d1128 = UsbX + 3.1 mm"
equation "d1134 = UsbZ - 2.3 mm"
equation "d1136 = UsbX - 5.1 mm"
equation "d1142 = UsbZ + 5.2 mm"
equation "d1144 = UsbX - 12.9 mm"
equation "d1150 = UsbZ + 6 mm"
equation "d1152 = UsbX - 10 mm"
equation "d1158 = UsbZ - 0.3 mm"
equation "d1160 = UsbX - 5.1 mm"
equation "d1166 = UsbZ + 2.3 mm"
equation "d1168 = UsbX - 5.1 mm"
equation "d1174 = UsbZ + 2.3 mm"
equation "d1176 = UsbX + 3.1 mm"
equation "d1182 = UsbZ + 0.3 mm"
equation "d1184 = UsbX - 5.1 mm"
equation "d1190 = UsbZ + 5.1 mm"
equation "d1192 = UsbX - 9.25 mm"
equation "d1197 = UsbZ + 5.1 mm"
equation "d1199 = UsbX + 9.25 mm"
equation "d1204 = UsbZ - 0.3 mm"
equation "d1206 = UsbX - 8 mm"
equation "d1212 = UsbZ - 0.4 mm"
equation "d1214 = UsbX - 8.1 mm"
equation "d1220 = UsbZ - 0.4 mm"
equation "d1222 = UsbX + 6.3 mm"
equation "d1228 = UsbZ - 0.4 mm"
equation "d1230 = UsbX - 4.63 mm"
equation "d1236 = UsbZ - 0.4 mm"
equation "d1238 = UsbX - 9.25 mm"
equation "d1243 = UsbZ - 0.4 mm"
equation "d1245 = UsbX + 9.25 mm"
equation "d1252 = UsbX - ( 4.17 mm )"
equation "d1253 = -( -( ( UsbZ - ( 1.63 mm ) ) + ( 3.26 mm ) ) )"
equation "d1262 = UsbX - ( 4.17 mm )"
equation "d1263 = -( -( ( UsbZ - ( 1.28 mm ) ) + ( 2.56 mm ) ) )"
equation "d1272 = UsbX - ( 3.97 mm )"
equation "d1273 = -( -( ( UsbZ - ( 1.43 mm ) ) + ( 2.86 mm ) ) )"
equation "d1282 = UsbX - ( 3.97 mm )"
equation "d1283 = -( -( ( UsbZ - ( 1.08 mm ) ) + ( 2.16 mm ) ) )"
equation "d1290 = UsbZ + 0.3 mm"
equation "d1292 = UsbX - 5.65 mm"
equation "d1298 = UsbZ + 0.3 mm"
equation "d1300 = UsbX + 4.12 mm"
equation "d1306 = UsbZ + 0.3 mm"
equation "d1308 = UsbX - 5.65 mm"
equation "d1314 = UsbZ + 0.3 mm"
equation "d1316 = UsbX + 4.12 mm"
equation "d1324 = UsbX - ( 3.9 mm )"
equation "d1325 = -( -( ( UsbZ - ( 1.05 mm ) ) + ( 2.1 mm ) ) )"
equation "d1332 = UsbZ - 0.35 mm"
equation "d1334 = UsbX - 3.345 mm"
equation "d1342 = UsbX - ( 4.75 mm )"
equation "d1343 = -( -( ( UsbZ - ( 1.86 mm ) ) + ( 3.72 mm ) ) )"
equation "d1352 = UsbX - ( 4.19 mm )"
equation "d1353 = -( -( ( UsbZ - ( 1.3 mm ) ) + ( 2.6 mm ) ) )"
equation "d1360 = UsbZ - 0.38 mm"
equation "d1362 = UsbX + ( -1.875 mm )"
equation "d1368 = UsbZ - 0.38 mm"
equation "d1370 = UsbX + ( -1.375 mm )"
equation "d1376 = UsbZ - 0.38 mm"
equation "d1378 = UsbX + ( -0.875 mm )"
equation "d1384 = UsbZ - 0.38 mm"
equation "d1386 = UsbX + ( -0.375 mm )"
equation "d1392 = UsbZ - 0.38 mm"
equation "d1394 = UsbX + ( 0.125 mm )"
equation "d1400 = UsbZ - 0.38 mm"
equation "d1402 = UsbX + ( 0.625 mm )"
equation "d1408 = UsbZ - 0.38 mm"
equation "d1410 = UsbX + ( 1.125 mm )"
equation "d1416 = UsbZ - 0.38 mm"
equation "d1418 = UsbX + ( 1.625 mm )"
equation "d1424 = UsbZ + 0.35 mm"
equation "d1426 = UsbX + ( -1.875 mm )"
equation "d1432 = UsbZ + 0.35 mm"
equation "d1434 = UsbX + ( -1.375 mm )"
equation "d1440 = UsbZ + 0.35 mm"
equation "d1442 = UsbX + ( -0.875 mm )"
equation "d1448 = UsbZ + 0.35 mm"
equation "d1450 = UsbX + ( -0.375 mm )"
equation "d1456 = UsbZ + 0.35 mm"
equation "d1458 = UsbX + ( 0.125 mm )"
equation "d1464 = UsbZ + 0.35 mm"
equation "d1466 = UsbX + ( 0.625 mm )"
equation "d1472 = UsbZ + 0.35 mm"
equation "d1474 = UsbX + ( 1.125 mm )"
equation "d1480 = UsbZ + 0.35 mm"
equation "d1482 = UsbX + ( 1.625 mm )"
equation "d1490 = UsbX - ( 7.2 mm )"
equation "d1491 = -( -( ( UsbZ - ( 4.2 mm ) ) + ( 8.4 mm ) ) )"
equation "d1498 = UsbZ - 9 mm"
equation "d1500 = UsbX - 13.1 mm"
equation "d1506 = UsbZ + 5.2 mm"
equation "d1508 = UsbX - 5.1 mm"
equation "d1512 = CaseDepth - Cover + CoverGap - ( UsbZ + 5.2 mm ) + 0.1 mm"
equation "d1514 = UsbZ + 7.7 mm"
equation "d1516 = UsbX - 5.1 mm"
equation "d1520 = CaseDepth - Cover + CoverGap - ( UsbZ + 7.7 mm ) + 0.1 mm"
equation "d1525 = CaseHeight - 50 mm"
equation "d1526 = CaseWidth - 53 mm"
equation "d1528 = CaseDepth - 10 mm"
equation "d1533 = CaseHeight - 19.5 mm"
equation "d1534 = CaseWidth - 25.5 mm"
equation "d1536 = CaseDepth - 10 mm"
equation "d1538 = CaseWidth - 17 mm"
equation "d1540 = -( -( GasZ ) )"
equation "d1541 = CaseHeight - 15 mm"
equation "d1545 = GasY"
equation "d1547 = CaseWidth - 14.25 mm"
equation "d1548 = -( -( GasZ ) )"
equation "d1552 = CaseWidth - 14.25 mm"
equation "d1554 = -( -( GasZ ) )"
equation "d1555 = GasY"
equation "d1562 = CaseHeight - 48 mm"
equation "d1563 = CaseWidth - 57 mm"
equation "d1565 = CaseDepth"
equation "d1570 = CaseHeight - 17.5 mm"
equation "d1571 = CaseWidth - 29.5 mm"
equation "d1573 = CaseDepth"
equation "d1578 = CaseHeight - 22 mm"
equation "d1579 = CaseWidth - 62.65 mm"
equation "d1581 = CaseDepth - 11.9 mm"
equation "d1586 = CaseHeight - 17.5 mm"
equation "d1589 = CaseDepth - 11.9 mm"
equation "d1594 = CaseHeight - 31 mm"
equation "d1595 = CaseWidth - 62.65 mm"
equation "d1597 = CaseDepth - 36 mm"
equation "d1602 = CaseHeight - 17.6 mm"
equation "d1605 = CaseDepth - 35 mm"
equation "d1607 = CaseWidth - 14.35 mm"
equation "d1609 = -( -( GasZ ) )"
equation "d1610 = GasY"
equation "d1614 = GasY - 0.1 mm"
equation "d1616 = CaseWidth - 14.25 mm"
equation "d1617 = -( -( GasZ ) )"
equation "d1621 = CaseWidth - 17.1 mm"
equation "d1623 = -( -( GasZ ) )"
equation "d1624 = CaseHeight - 15 mm"
equation "d1630 = -( -( GasZ ) )"
equation "d1631 = GasY"
equation "d1638 = GasY"
equation "d1642 = CaseHeight - 34.6 mm"
equation "d1645 = -( -( 33.5 mm ) )"
equation "d1649 = CaseWidth - 52.1 mm"
equation "d1651 = -( -( 21.75 mm ) )"
equation "d1652 = CaseHeight - 37.5 mm"
equation "d1656 = CaseDepth - 13 mm"
equation "d1659 = CaseHeight - 21 mm"
equation "d1663 = CaseDepth - 11 mm"
equation "d1666 = CaseHeight - 21 mm"
equation "d1670 = CaseDepth - 13 mm"
equation "d1672 = CaseWidth - 54.5 mm"
equation "d1673 = CaseHeight - 45 mm"
equation "d1677 = CaseDepth - 11 mm"
equation "d1679 = CaseWidth - 54.5 mm"
equation "d1680 = CaseHeight - 45 mm"
equation "d1684 = CaseDepth - 13 mm"
equation "d1687 = CaseHeight - 7.8 mm"
equation "d1691 = CaseDepth - 11 mm"
equation "d1694 = CaseHeight - 7.8 mm"
equation "d1698 = CaseDepth - 13 mm"
equation "d1700 = CaseWidth - 17 mm"
equation "d1701 = CaseHeight - 7.8 mm"
equation "d1705 = CaseDepth - 11 mm"
equation "d1707 = CaseWidth - 17 mm"
equation "d1708 = CaseHeight - 7.8 mm"
equation "d1712 = CaseHeight - 50 mm"
equation "d1715 = -( -( 31.5 mm ) )"
equation "d1719 = CaseHeight - 50.1 mm"
equation "d1722 = -( -( 31.5 mm ) )"
equation "d1726 = CaseDepth - 7 mm"
equation "d1729 = CaseHeight - 50 mm"
equation "d1730 = CaseWidth - 53 mm"
equation "d1734 = CaseDepth - 7 mm"
equation "d1737 = CaseHeight - 19.5 mm"
equation "d1738 = CaseWidth - 25.5 mm"
equation "d1742 = CaseDepth - 7.1 mm"
equation "d1745 = CaseHeight - 21 mm"
equation "d1749 = CaseDepth - 7.1 mm"
equation "d1751 = CaseWidth - 54.5 mm"
equation "d1752 = CaseHeight - 45 mm"
equation "d1756 = CaseDepth - 7.1 mm"
equation "d1759 = CaseHeight - 7.8 mm"
equation "d1763 = CaseDepth - 7.1 mm"
equation "d1765 = CaseWidth - 17 mm"
equation "d1766 = CaseHeight - 7.8 mm"
equation "d1770 = CaseWidth - 50 mm"
equation "d1772 = -( -( 21.75 mm ) )"
equation "d1773 = CaseHeight - 37.5 mm"
equation "d1777 = CaseWidth - 50.1 mm"
equation "d1779 = -( -( 21.75 mm ) )"
equation "d1780 = CaseHeight - 37.5 mm"
equation "d1784 = CaseWidth - 46 mm"
equation "d1786 = -( -( 21.75 mm ) )"
equation "d1787 = CaseHeight - 37.5 mm"
equation "d1791 = CaseWidth - 52.5 mm"
equation "d1793 = -( -( 21.75 mm ) )"
equation "d1794 = CaseHeight - 37.5 mm"
equation "d1800 = CaseWidth - 14.25 mm"
equation "d1801 = CaseHeight - 42.5 mm"
equation "d1809 = CaseHeight - 47.7 mm"
equation "d1816 = -( -( 16.6 mm ) )"
equation "d1817 = CaseHeight - 35 mm"
equation "d1824 = CaseHeight - 45.7 mm"
equation "d1832 = CaseHeight - 17 mm"
equation "d1839 = -( -( 13 mm ) )"
equation "d1840 = CaseHeight - 15.8 mm"
equation "d1846 = -( -( 24 mm ) )"
equation "d1847 = CaseHeight - 15.8 mm"
equation "d1853 = -( -( 13 mm ) )"
equation "d1854 = CaseHeight - 8.7 mm"
equation "d1860 = -( -( 24 mm ) )"
equation "d1861 = CaseHeight - 8.7 mm"
equation "d1867 = CaseWidth - 32 mm"
equation "d1868 = CaseHeight - 17.2 mm"
equation "d1875 = CaseWidth - 20 mm"
equation "d1876 = CaseHeight - 10 mm"
equation "d1883 = CaseWidth - 30 mm"
equation "d1884 = CaseHeight - 15 mm"
equation "d1889 = CaseWidth - 3 mm"
equation "d1891 = -( -( GasZ ) )"
equation "d1892 = GasY"
equation "d1896 = ( CaseWidth - 3 mm ) - 0.1 mm"
equation "d1898 = -( -( GasZ ) )"
equation "d1899 = GasY"
equation "d1901 = ( 9 mm ) + 0.2 mm"
equation "d1905 = -( -( GasZ ) )"
equation "d1906 = GasY"
equation "d1910 = ( -6 mm ) - 0.1 mm"
equation "d1912 = -( -( GasZ ) )"
equation "d1913 = GasY"
equation "d1915 = ( 9 mm ) + 0.2 mm"
equation "d1917 = CaseWidth - 46.2 mm"
equation "d1919 = -( -( 21.75 mm ) )"
equation "d1920 = CaseHeight - 37.5 mm"
equation "d1924 = CaseWidth - 46.3 mm"
equation "d1926 = -( -( 21.75 mm ) )"
equation "d1927 = CaseHeight - 37.5 mm"
equation "d1931 = CaseHeight - 51.3 mm"
equation "d1934 = -( -( 31.5 mm ) )"
equation "d1940 = CaseDepth - 1.65 mm"
equation "d1948 = CaseDepth - 4 mm"
equation "d1954 = CaseWidth - 9 mm"
equation "d1956 = PcbZ + 1.6 mm"
equation "d1962 = CaseWidth - 9 mm"
equation "d1970 = CaseWidth - 16 mm"
equation "d1978 = CaseWidth - 8 mm"
equation "d1980 = CaseDepth - 1.65 mm"
equation "d1987 = CaseHeight - 8 mm"
equation "d1988 = CaseDepth - 1.65 mm"
equation "d1994 = CaseWidth - 8 mm"
equation "d1995 = CaseHeight - 8 mm"
equation "d1996 = CaseDepth - 1.65 mm"
equation "d2002 = CaseWidth - 8 mm"
equation "d2004 = CaseDepth - 4 mm"
equation "d2011 = CaseHeight - 8 mm"
equation "d2012 = CaseDepth - 4 mm"
equation "d2018 = CaseWidth - 8 mm"
equation "d2019 = CaseHeight - 8 mm"
equation "d2020 = CaseDepth - 4 mm"
equation "d2028 = PcbZ + 1.6 mm"
equation "d2042 = DisplayX + 2.65 mm"
equation "d2050 = CaseWidth - 16 mm"
equation "d2058 = DisplayX + 2.65 mm"
equation "d2066 = UsbX - 9.25 mm"
equation "d2068 = UsbZ + 7.2 mm"
equation "d2074 = UsbX + 9.25 mm"
equation "d2076 = UsbZ + 7.2 mm"
equation "d2082 = UsbX - 9.25 mm"
equation "d2084 = UsbZ + 5.2 mm"
equation "d2090 = UsbX + 9.25 mm"
equation "d2092 = UsbZ + 5.2 mm"
equation "d2099 = CaseHeight - 21 mm"
equation "d2100 = CaseDepth - 5 mm"
equation "d2106 = CaseWidth - 54.5 mm"
equation "d2107 = CaseHeight - 45 mm"
equation "d2108 = CaseDepth - 5 mm"
equation "d2115 = CaseHeight - 7.8 mm"
equation "d2116 = CaseDepth - 5 mm"
equation "d2122 = CaseWidth - 17 mm"
equation "d2123 = CaseHeight - 7.8 mm"
equation "d2124 = CaseDepth - 5 mm"
equation "d2131 = CaseHeight - 21 mm"
equation "d2132 = CaseDepth - 7 mm"
equation "d2138 = CaseWidth - 54.5 mm"
equation "d2139 = CaseHeight - 45 mm"
equation "d2140 = CaseDepth - 7 mm"
equation "d2147 = CaseHeight - 7.8 mm"
equation "d2148 = CaseDepth - 7 mm"
equation "d2154 = CaseWidth - 17 mm"
equation "d2155 = CaseHeight - 7.8 mm"
equation "d2156 = CaseDepth - 7 mm"
equation "d2162 = GasZ"
equation "d2164 = CaseWidth - 14.25 mm"
equation "d2165 = GasY"
equation "d2168 = GasZ"
equation "d2170 = CaseWidth - 14.25 mm"
equation "d2171 = CaseHeight - 15 mm"
equation "d2174 = GasZ"
equation "d2176 = CaseWidth - 14.25 mm"
equation "d2177 = GasY"
equation "d2180 = GasZ"
equation "d2182 = CaseWidth - 14.25 mm"
equation "d2183 = CaseHeight - 15 mm"
equation "d2189 = GasY"
equation "d2195 = GasY"
equation "d2198 = CaseWidth - 14.35 mm"
equation "d2200 = -( -( GasZ ) )"
equation "d2201 = GasY"
equation "d2205 = GasY - 0.1 mm"
equation "d2207 = CaseWidth - 14.25 mm"
equation "d2208 = -( -( GasZ ) )"
equation "d2212 = CaseWidth - 20.1 mm"
equation "d2214 = -( -( GasZ ) )"
equation "d2215 = CaseHeight - 15 mm"
equation "d2222 = CaseHeight - 46 mm"
equation "d2230 = CaseHeight - 28 mm"
equation "d2238 = CaseHeight - 12 mm"
equation "d2246 = CaseHeight - 52.5 mm"
equation "d2247 = CaseWidth - 50 mm - 25 mm"
equation "d2249 = CaseDepth - 7.5 mm"
equation "d2253 = CaseWidth - 49.5 mm"
equation "d2254 = CaseHeight - 50 mm"
equation "d2257 = CaseDepth - 7.5 mm"
equation "d2262 = CaseHeight - 12.5 mm"
equation "d2267 = CaseDepth - 4.8 mm"
equation "d2270 = CaseHeight - 46 mm"
equation "d2273 = 4.9 mm - Cover + CoverGap"
equation "d2275 = CaseDepth - 4.8 mm"
equation "d2278 = CaseHeight - 30 mm"
equation "d2281 = 4.9 mm - Cover + CoverGap"
equation "d2283 = CaseDepth - 4.8 mm"
equation "d2286 = CaseHeight - 14 mm"
equation "d2289 = 4.9 mm - Cover + CoverGap"
equation "d2294 = CaseHeight - 47 mm"
equation "d2302 = CaseHeight - 25 mm"
equation "d2310 = CaseHeight - 47 mm"
equation "d2318 = CaseHeight - 24.5 mm"
equation "d2326 = CaseHeight - 48.5 mm"
equation "d2334 = CaseHeight - 16 mm"
equation "d2342 = CaseHeight - 16 mm"
equation "d2345 = CaseDepth - 34.2 mm"
equation "d2350 = CaseHeight - 10.2 mm"
equation "d2358 = CaseHeight - 10.2 mm"
equation "d2361 = CaseDepth - 34.2 mm"
equation "d2366 = CaseHeight - 16.5 mm"
equation "d2374 = CaseHeight - 16.5 mm"
equation "d2381 = CaseWidth - 31 mm"
equation "d2382 = CaseHeight - 16 mm"
equation "d2389 = CaseWidth - 18 mm"
equation "d2390 = CaseHeight - 8 mm"
equation "d2397 = CaseWidth - 17 mm"